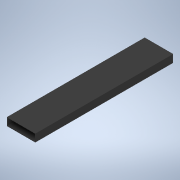
# Autodesk Inventor part: RubberPiece
Saved by Autodesk Inventor 2020.2 (Build 242310000, 310)
## iProperties
Created: 2021-07-19
Part Number: RubberPiece
Material: Generic
Document SubType Name: Modeling
Designer: JK
Density: 1 g/cm^3
Appearance: Rubber - Black
Author: JK
Autodesk Inventor part; units mm, degrees
ref_plane "YZ Plane" through (0, 0, 0) normal (1, 0, 0) x (0, 1, 0)
ref_plane "XZ Plane" through (0, 0, 0) normal (0, 1, 0) x (-1, 0, 0)
ref_plane "XY Plane" through (0, 0, 0) normal (0, 0, 1) x (1, 0, 0)
sketch "Sketch1" plane through (0, 0, 0) normal (0, 1, 0) x (-1, 0, 0)
  line L0 (-10.3, 50) -> (10.3, 50)
  line L1 (10.3, 50) -> (10.3, -50)
  line L2 (10.3, -50) -> (-10.3, -50)
  line L3 (-10.3, -50) -> (-10.3, 50)
  line L4 (-10.3, 50) -> (10.3, -50) construction
  line L5 (10.3, 50) -> (-10.3, -50) construction
  point P0 (0, 0)
  dimension "d0" = 100
  dimension "d1" = 20.6
  constraints: 12 end point, 2 midpoint, 2 parallel, 1 horizontal, 1 perpendicular
  measures "d0" distance of L0.end L1.end
  measures "d1" distance of L1.end L2.end
extrude "Extrusion1" add sketch "Sketch1" along normal blind 5.6
sketch "Sketch2" plane through (-10.3, 0, 50) normal (0, 0, 1) x (1, 0, 0)
  line L0 (0.3, 0.3) -> (20.3, 0.3)
  line L1 (20.3, 0.3) -> (20.3, 5.3)
  line L2 (20.3, 5.3) -> (0.3, 5.3)
  line L3 (0.3, 5.3) -> (0.3, 0.3)
  line L4 (0, 0) -> (20.6, 0) projected
  line L5 (0, 5.6) -> (20.6, 5.6) projected
  line L6 (20.6, 0) -> (20.6, 5.6) projected
  line L7 (0, 0) -> (0, 5.6) projected
  point P0 (10.3, 0)
  dimension "d4" = 0.3
  dimension "d5" = 0.3
  dimension "d6" = 0.3
  dimension "d7" = 0.3
  constraints: 8 end point, 2 parallel, 1 horizontal, 1 perpendicular
  measures "d4" distance between parallel lines of L4 L0
  measures "d5" distance between parallel lines of L5 L2
  measures "d6" distance between parallel lines of L6 L1
  measures "d7" distance between parallel lines of L7 L3
extrude "Extrusion2" cut sketch "Sketch2" against normal through all contours L3 L2 L1 L0
fillet "Fillet1" radius 0.05 4 edges at (-10.3, 5.6, 0) (-10.3, 0, 0) (10, 5.3, 0) (10.3, 0, 0)
body "Solid1"
